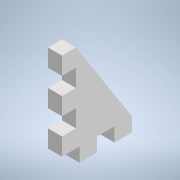
# Autodesk Inventor part: laterali
Saved by Autodesk Inventor 2020.2 (Build 242310000, 310)
## iProperties
Created: 2020-02-13
Part Number: laterali
Material: Generico
Document SubType Name: Modeling
Designer: socci
Density: 1 g/cm^3
Appearance: Giallo
Author: socci
Autodesk Inventor part; units mm, degrees
ref_plane "YZ Plane" through (0, 0, 0) normal (1, 0, 0) x (0, 1, 0)
ref_plane "XZ Plane" through (0, 0, 0) normal (0, 1, 0) x (-1, 0, 0)
ref_plane "XY Plane" through (0, 0, 0) normal (0, 0, 1) x (1, 0, 0)
sketch "Schizzo1" plane through (0, 0, 0) normal (1, 0, 0) x (0, 1, 0)
  line L0 (0, 0) -> (25, 0)
  line L1 (25, 0) -> (0, -16)
  line L2 (0, -16) -> (0, 0)
  dimension "d0" = 16
  dimension "d1" = 25
  constraints: 6 end point, 1 horizontal, 1 perpendicular
  measures "d0" distance of L1.end L0.start
  measures "d1" distance of L0.start L0.end
extrude "Estrusione1" add sketch "Schizzo1" along normal blind 4
sketch "Schizzo2" plane through (4, 0, 0) normal (1, 0, 0) x (0, 0, -1)
  line L0 (0, 0) -> (16, 0) projected
  line L1 (16, 0) -> (11, 0)
  line L2 (11, 0) -> (11, -4)
  line L3 (11, -4) -> (16, -4)
  line L4 (16, -4) -> (16, 0)
  line L5 (11, 0) -> (6, 0)
  line L6 (6, 0) -> (1, 0)
  line L7 (1, 0) -> (1, -4)
  line L8 (1, -4) -> (6, -4)
  line L9 (6, -4) -> (6, 0)
  line L10 (0, 25) -> (0, 0) projected
  line L11 (0, 0) -> (0, 5)
  line L12 (0, 5) -> (-4, 5)
  line L13 (-4, 5) -> (-4, 0)
  line L14 (-4, 0) -> (0, 0)
  line L15 (0, 15) -> (-4, 15)
  line L16 (-4, 15) -> (-4, 10)
  line L17 (-4, 10) -> (0, 10)
  line L18 (0, 10) -> (0, 15)
  line L19 (0, 25) -> (-4, 25)
  line L20 (-4, 25) -> (-4, 20)
  line L21 (-4, 20) -> (0, 20)
  line L22 (0, 20) -> (0, 25)
  dimension "d4" = 5
  dimension "d5" = 4
  dimension "d6" = 5
  dimension "d7" = 5
  dimension "d8" = 4
  dimension "d9" = 5
  dimension "d10" = 4
  dimension "d13" = 10
  constraints: 42 end point, 6 parallel, 4 point on line, 3 perpendicular, 1 vertical, 16 other
  measures "d4" distance of L0.end L1.end
  measures "d5" distance of L2.end L1.end
  measures "d6" distance of L1.end L5.end
  measures "d7" distance of L5.end L6.end
  measures "d8" distance of L7.end L6.end
  measures "d9" distance of L0.start L11.end
  measures "d10" distance of L12.end L11.end
  measures "d13" distance of L11.end L15.start
extrude "Estrusione2" add sketch "Schizzo2" against normal blind 4
